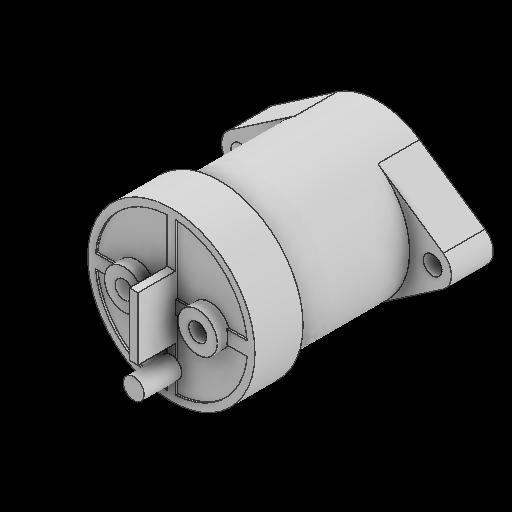
# Autodesk Inventor part: HiitioContactor
Saved by Autodesk Inventor 2025.2 (Build 292293000, 293)
## iProperties
Created: 2026-05-17
Part Number: HiitioContactor
Material: Generic
Document SubType Name: Modeling
Designer: valer
Density: 1 g/cm^3
Appearance: Default
Author: valer
Autodesk Inventor part; units mm, degrees
ref_plane "YZ Plane" through (0, 0, 0) normal (1, 0, 0) x (0, 1, 0)
ref_plane "XZ Plane" through (0, 0, 0) normal (0, 1, 0) x (-1, 0, 0)
ref_plane "XY Plane" through (0, 0, 0) normal (0, 0, 1) x (1, 0, 0)
sketch "Base" plane through (0, 0, 0) normal (0, 0, 1) x (1, 0, 0)
  circle A0 centre (0, 0) radius 17.5
  circle A1 centre (23, 0) radius 2.25
  line L0 (-38.5, 0) -> (38.5, 0) construction
  line L1 (0, -24.5) -> (0, 24.5) construction
  circle A2 centre (-23, 0) radius 2.25
  circle A3 centre (23, 0) radius 4.5
  circle A4 centre (-23, 0) radius 4.5
  line L2 (-27.5, 0) -> (27.5, 0) construction
  line L3 (9.8913, 14.4365) -> (25.5435, 3.7122)
  line L4 (25.5435, -3.7122) -> (9.8913, -14.4365)
  line L5 (-25.5435, 3.7122) -> (-9.8913, 14.4365)
  line L6 (-25.5435, -3.7122) -> (-9.8913, -14.4365)
  dimension "d0" = 35
  dimension "d1" = 4.5
  dimension "d2" = 2.25
  dimension "d3" = 46
  dimension "d4" = 55
  constraints: 10 end point, 10 point on circle, 8 tangent, 5 centre point, 3 coincident, 3 point on line, 1 equal radius, 1 symmetric about line, 1 other
  measures "d0" diameter of A0
  measures "d1" diameter of A1
  measures "d2" radial gap between concentric circles of A3 A1
  measures "d3" distance of A1.centre A2.centre
  measures "d4" distance of L2.end L2.start
extrude "BaseFeature" add sketch "Base" along normal blind 10
sketch "Body" plane through (0, 0, 10) normal (0, 0, 1) x (1, 0, 0)
  circle A0 centre (0, 0) radius 17.5
  arc A1 (-9.8913, -14.4365) -> (9.8913, -14.4365) centre (0, 0) ccw projected
  constraints: 1 centre point, 1 coincident, 1 concentric
extrude "BodyFeature" add sketch "Body" along normal blind 28
sketch "Head" plane through (0, 0, 38) normal (0, 0, 1) x (1, 0, 0)
  circle A0 centre (0, 0) radius 20
  dimension "d9" = 40
  constraints: 1 centre point, 1 coincident
  measures "d9" diameter of A0
extrude "HeadFeature" add sketch "Head" along normal blind 11.5
sketch "Top" plane through (0, 0, 49.5) normal (0, 0, 1) x (1, 0, 0)
  circle A0 centre (0, 0) radius 18.2
  circle A1 centre (0, 0) radius 20 projected
  dimension "d12" = 1.8
  constraints: 1 centre point, 1 coincident
  measures "d12" radial gap between concentric circles of A1 A0
extrude "TopFeature" cut sketch "Top" against normal blind 0.5 contours A0
sketch "Sketch5" plane through (0, 0, 49) normal (0, 0, 1) x (1, 0, 0)
  line L0 (-38.5, 0) -> (38.5, 0) construction
  circle A0 centre (8.8, 0) radius 4.7
  line L1 (0, -28) -> (0, 28) construction
  circle A1 centre (-8.8, 0) radius 4.7
  line L2 (8.8, 0) -> (13.5, 0) construction
  line L3 (-8.8, 0) -> (-13.5, 0) construction
  point P0 (0, 0)
  dimension "d15" = 9.4
  dimension "d16" = 27
  constraints: 4 end point, 3 point on line, 2 horizontal alignment, 1 symmetric about line, 1 vertical, 4 other
  measures "d16" distance of L2.end L3.end
extrude "Extrusion5" add sketch "Sketch5" along normal blind 3
sketch "Sketch6" plane through (8.8, 0, 52) normal (0, 0, 1) x (1, 0, 0)
  circle A0 centre (0, 0) radius 4.7 projected
  circle A1 centre (-17.6, 0) radius 4.7 projected
  circle A2 centre (-17.6, 0) radius 4.7 projected
  circle A3 centre (-17.6, 0) radius 2.15
  circle A4 centre (0, 0) radius 2.15
  point P0 (-8.8, 0)
  dimension "d19" = 4.3
  constraints: 2 centre point, 2 coincident, 1 equal radius
  measures "d19" diameter of A3
extrude "Extrusion6" cut sketch "Sketch6" against normal blind 6 contours A3 | A4
sketch "Sketch7" plane through (0, 0, 49) normal (0, 0, 1) x (1, 0, 0)
  circle A0 centre (-8.8, 0) radius 4.7 projected
  circle A1 centre (8.8, 0) radius 4.7 projected
  circle A2 centre (0, 0) radius 18.2 projected
  line L0 (-18.2, 1.625) -> (18.2, 1.625)
  line L1 (18.2, 1.625) -> (18.2, -1.625)
  line L2 (18.2, -1.625) -> (-18.2, -1.625)
  line L3 (-18.2, -1.625) -> (-18.2, 1.625)
  line L4 (-38.5, 0) -> (38.5, 0) construction
  circle A3 centre (0, 0) radius 18.2 projected
  point P0 (-18.2, 0)
  point P1 (13.2101, -1.625)
  point P2 (18.1273, -1.625)
  point P3 (18.1273, 1.625)
  point P4 (13.2101, 1.625)
  point P5 (-4.3899, -1.625)
  point P6 (4.3899, -1.625)
  point P7 (4.3899, 1.625)
  point P8 (-4.3899, 1.625)
  point P9 (-18.1273, -1.625)
  point P10 (-13.2101, -1.625)
  point P11 (-13.2101, 1.625)
  point P12 (-18.1273, 1.625)
  dimension "d22" = 3.25
  constraints: 8 end point, 2 parallel, 1 horizontal, 1 horizontal alignment, 1 midpoint, 1 perpendicular, 1 point on line, 1 vertical, 1 other
  measures "d22" distance between parallel lines of L2 L0
extrude "Extrusion7" add sketch "Sketch7" along normal up to surface (0.5 mm away) contours A0 L0 A1 L2 | A0 L2 A2 L0 | L0 A2 L2 A1
sketch "Sketch8" plane through (0, 0, 49) normal (0, 0, 1) x (1, 0, 0)
  line L0 (0, -28) -> (0, 28) construction
  line L1 (-1, 18.2) -> (1, 18.2)
  line L2 (1, 18.2) -> (1, -18.2)
  line L3 (1, -18.2) -> (-1, -18.2)
  line L4 (-1, -18.2) -> (-1, 18.2)
  arc A0 (18.1273, 1.625) -> (-18.1273, 1.625) centre (0, 0) ccw projected
  arc A1 (-18.1273, -1.625) -> (18.1273, -1.625) centre (0, 0) ccw projected
  point P0 (0, 18.2)
  dimension "d25" = 2
  constraints: 8 end point, 2 parallel, 2 tangent, 1 horizontal, 1 midpoint, 1 perpendicular, 1 point on line
  measures "d25" distance between parallel lines of L2 L4
extrude "Extrusion8" add sketch "Sketch8" along normal up to surface (0.5 mm away)
sketch "Sketch9" plane through (0, 0, 49.5) normal (0, 0, 1) x (1, 0, 0)
  line L0 (0, -28) -> (0, 28) construction
  circle A0 centre (0, -12.8363) radius 2.5
  line L1 (-1, 1.625) -> (-1, 18.1725) projected
  line L2 (1, -1.625) -> (1, -18.1725) projected
  line L3 (-1, 7.5) -> (1, 7.5)
  line L4 (1, 7.5) -> (1, -7.5)
  line L5 (1, -7.5) -> (-1, -7.5)
  line L6 (-1, -7.5) -> (-1, 7.5)
  line L7 (-38.5, 0) -> (38.5, 0) construction
  line L8 (0, -7.5) -> (0, -18.1725) construction
  point P0 (0, 0)
  point P1 (1, 0)
  dimension "d28" = 5
  dimension "d29" = 15
  dimension "d30" = 5.3362
  dimension "d31" = 5.3362
  constraints: 10 end point, 5 point on line, 3 midpoint, 2 parallel, 1 centre point, 1 horizontal, 1 perpendicular
  measures "d28" diameter of A0
  measures "d29" distance between parallel lines of L5 L3
  measures "d30" distance from line of L5 A0.centre
  measures "d31" vertical distance of L2.end A0.centre
extrude "Extrusion9" add sketch "Sketch9" along normal blind 9
equation "\"d26\" = d25"
body "Solid1"
